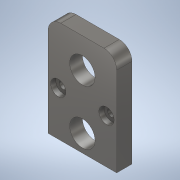
# Autodesk Inventor part: kicker_base_v2
Saved by Autodesk Inventor 2020 (Build 240168000, 168)
## iProperties
Part Number: kicker_base_v2
Material: Steel, Carbon
Document SubType Name: Modeling
Designer: rYan
Density: 7.85 g/cm^3
Appearance: Semi-Polished
Mass: 13.4819 g
Surface Area: 35.0889 cm^2
Volume: 4.99329 cm^3
Author: rYan
Autodesk Inventor part; units mm, degrees
ref_plane "YZ Plane" through (0, 0, 0) normal (1, 0, 0) x (0, 1, 0)
ref_plane "XZ Plane" through (0, 0, 0) normal (0, 1, 0) x (-1, 0, 0)
ref_plane "XY Plane" through (0, 0, 0) normal (0, 0, 1) x (1, 0, 0)
sketch "Skizze1" plane through (0, 0, 0) normal (0, 1, 0) x (-1, 0, 0)
  line L0 (13.5, 0) -> (-13.5, 0)
  line L1 (-13.5, 0) -> (-13.5, 40)
  line L2 (-13.5, 40) -> (13.5, 40)
  line L3 (13.5, 40) -> (13.5, 0)
  line L4 (0, -12.8) -> (0, 48.8) projected
  circle A0 centre (0, 6.75) radius 5
  circle A1 centre (0, 28.25) radius 5
  circle A2 centre (0, 28.25) radius 10.75 construction
  circle A3 centre (0, 6.75) radius 10.75 construction
  line L5 (0, 6.75) -> (0, -4) construction
  point P0 (0, 0)
  dimension "d4" = 21.5
  dimension "d0" = 27
  dimension "d1" = 10
  dimension "d2" = 10
  dimension "d3" = 21.5
  dimension "d8" = 4
  dimension "d35" = 40
  constraints: 10 end point, 3 centre point, 3 point on line, 2 coincident, 2 parallel, 1 horizontal, 1 midpoint, 1 perpendicular, 1 vertical alignment, 4 other
  measures "d0" distance of L1.end L2.end
  measures "d1" diameter of A0
  measures "d2" diameter of A1
  measures "d3" diameter of A2
  measures "d8" distance from line of L0 L5.end
  measures "d35" distance of L0.end L1.end
extrude "Extrusion1" add sketch "Skizze1" along normal blind 6 contours L0 L4 A0 A1 L2 L3 | L0 L1 L2 L4 A1 A0
sketch "Skizze2" plane through (13.5, 0, 0) normal (0, 0, -1) x (-1, 0, 0)
  line L0 (0, 0) -> (27, 0) projected
  line L1 (0, 6) -> (27, 6) projected
  line L2 (25.041, 3) -> (0, 3) construction
  line L3 (13.5, 0) -> (13.5, 6) construction
  line L4 (27, 0) -> (27, 6) projected
  line L5 (0, 0) -> (0, 6) projected
  point P0 (23, 3)
  point P1 (4, 3)
  dimension "d68" = 9.5
  constraints: 4 end point, 2 midpoint, 2 point on line, 1 symmetric about line
  measures "d68" distance from line of L3 point (23, 3)
hole "Bohrung1" at (-9.5, 3, 0) at (9.5, 3, 0) direction (0, 0, 1) diameter 2.459 depth 8 tip angle 118 thread size "M3x0.5" class "6H" standard "ISO Metric profile"
sketch "Skizze5" plane through (0, 6, 0) normal (0, 1, 0) x (1, 0, 0)
  circle A0 centre (0, -28.25) radius 5 projected
  circle A1 centre (0, -28.25) radius 5 projected
  circle A2 centre (0, -6.75) radius 5 projected
  circle A3 centre (0, -6.75) radius 5 projected
  circle A4 centre (0, -28.25) radius 10.55
  circle A5 centre (0, -6.75) radius 10.55
  point P0 (0, 0)
  dimension "d44" = 21.1
  constraints: 2 centre point, 2 coincident, 1 equal radius
  measures "d44" diameter of A4
extrude "Extrusion2" cut sketch "Skizze5" against normal blind 1
fillet "Fillet2" radius 5 2 edges at (-13.5, 3, 40) (13.5, 3, 40)
sketch "Sketch7" plane through (0, 0, 0) normal (0, -1, 0) x (1, 0, 0)
  arc A0 (13.5, 35) -> (8.5, 40) centre (8.5, 35) ccw construction
  line L0 (-8.5, 40) -> (8.5, 40) construction
  arc A1 (-8.5, 40) -> (-13.5, 35) centre (-8.5, 35) ccw construction
  line L1 (-13.5, 0) -> (-13.5, 35) construction
  line L2 (13.5, 0) -> (-13.5, 0) construction
  line L3 (13.5, 35) -> (13.5, 0) construction
  circle A2 centre (0, 28.25) radius 5 construction
  circle A3 centre (0, 6.75) radius 5 construction
  line L4 (0, 28.25) -> (0, 6.75) construction
  line L5 (-13.5, 0) -> (-13.5, 35) construction
  line L6 (-13.5, 17.5) -> (13.5, 17.5) construction
  line L7 (13.5, 35) -> (13.5, 0) construction
  point P0 (0, 0)
  point P1 (0, 17.5)
  point P2 (-9.5, 17.5)
  point P3 (9.5, 17.5)
  dimension "d66" = 9.5
  dimension "d67" = 9.5
  constraints: 4 end point, 4 midpoint, 2 point on line, 1 perpendicular, 1 vertical
  measures "d66" distance from line of L4 point (9.5, 17.5)
  measures "d67" distance from line of point (-9.5, 17.5) L4
hole "Hole5" at (-9.5, 0, 17.5) at (9.5, 0, 17.5) direction (0, 1, 0) diameter 3.2 depth 8 tip angle 118 counterbore diameter 6 counterbore depth 2
equation "\"d4\" = d3"
equation "\"d67\" = d66"
